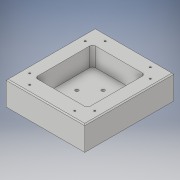
# Autodesk Inventor part: Chuck
Saved by Autodesk Inventor 2019.4 (Build 234330000, 330)
## iProperties
Created: 2020-11-12
Part Number: Chuck
Material: Generic
Document SubType Name: Modeling
Designer: caleb
Density: 1 g/cm^3
Appearance: Default
Author: caleb
Autodesk Inventor part; units mm, degrees
ref_plane "YZ Plane" through (0, 0, 0) normal (1, 0, 0) x (0, 1, 0)
ref_plane "XZ Plane" through (0, 0, 0) normal (0, 1, 0) x (-1, 0, 0)
ref_plane "XY Plane" through (0, 0, 0) normal (0, 0, 1) x (1, 0, 0)
sketch "Sketch1" plane through (0, 0, 0) normal (0, 1, 0) x (-1, 0, 0)
  line L0 (75, 85) -> (-75, 85)
  line L1 (-75, 85) -> (-75, -85)
  line L2 (-75, -85) -> (75, -85)
  line L3 (75, -85) -> (75, 85)
  point P0 (0, 0)
  dimension "d0" = 170
  dimension "d1" = 150
  dimension "d8" = 85
  dimension "d9" = 75
  constraints: 8 end point, 2 parallel, 1 horizontal, 1 perpendicular
  measures "d0" distance of L2.end L0.start
  measures "d1" distance of L0.start L0.end
  measures "d8" distance from line of L0 point (0, 0)
  measures "d9" distance from line of L3 point (0, 0)
extrude "Extrusion1" add sketch "Sketch1" along normal blind 46
sketch "Sketch2" plane through (0, 46, 0) normal (0, 1, 0) x (1, 0, 0)
  line L0 (-50, -55) -> (50, -55)
  line L1 (50, -55) -> (50, 55)
  line L2 (50, 55) -> (-50, 55)
  line L3 (-50, 55) -> (-50, -55)
  point P0 (0, 0)
  dimension "d4" = 100
  dimension "d5" = 110
  dimension "d6" = 55
  dimension "d7" = 50
  constraints: 8 end point, 2 parallel, 1 horizontal, 1 perpendicular
  measures "d4" distance of L0.start L0.end
  measures "d5" distance of L2.end L0.start
  measures "d6" distance from line of L0 point (0, 0)
  measures "d7" distance from line of L3 point (0, 0)
extrude "Extrusion2" cut sketch "Sketch2" against normal blind 36
fillet "Fillet1" radius 5 1 edges at (-50, 28, -55)
fillet "Fillet2" radius 5 1 edges at (-50, 28, 55)
fillet "Fillet3" radius 5 1 edges at (50, 28, 55)
fillet "Fillet4" radius 5 1 edges at (50, 28, -55)
chamfer "Chamfer1" distance 2 angle 45 4 edges at (75, 46, 0) (0, 46, -85) (0, 46, 85) (-75, 46, 0)
sketch "Sketch3" plane through (0, 46, 0) normal (0, 1, 0) x (1, 0, 0)
  circle A0 centre (43, -72) radius 2
  line L0 (73, -83) -> (-73, -83) projected
  line L1 (73, 83) -> (73, -83) projected
  circle A1 centre (62, -53) radius 2
  circle A2 centre (43, 72) radius 2
  circle A3 centre (62, 53) radius 2
  circle A4 centre (-43, -72) radius 2
  circle A5 centre (-62, -53) radius 2
  circle A6 centre (-43, 72) radius 2
  circle A7 centre (-62, 53) radius 2
  point P0 (0, 0)
  point P1 (-73, 83)
  dimension "d19" = 4
  dimension "d20" = 11
  dimension "d21" = 30
  dimension "d22" = 4
  dimension "d23" = 11
  dimension "d24" = 30
  constraints: 8 centre point
  measures "d19" diameter of A0
  measures "d20" distance from line of L0 A0.centre
  measures "d21" distance from line of L1 A0.centre
  measures "d22" diameter of A1
  measures "d23" distance from line of L1 A1.centre
  measures "d24" distance from line of L0 A1.centre
hole "Hole1" at (43, 46, -72) at (62, 46, -53) at (62, 46, 53) at (43, 46, 72) at (-43, 46, 72) at (-62, 46, 53) at (-62, 46, -53) at (-43, 46, -72) direction (0, -1, 0) diameter 3.242 depth 11.8 tip angle 118 thread size "M4x0.7" class "6H" standard "ISO Metric profile"
sketch "Sketch4" plane through (0, 10, 0) normal (0, 1, 0) x (1, 0, 0)
  circle A0 centre (-25, 0) radius 3
  circle A1 centre (0, 25) radius 3
  circle A2 centre (25, 0) radius 3
  circle A3 centre (0, -25) radius 3
  point P0 (0, 0)
  dimension "d32" = 6
  dimension "d34" = 25
  dimension "d35" = 6
  dimension "d36" = 6
  dimension "d37" = 6
  dimension "d39" = 25
  dimension "d40" = 25
  dimension "d42" = 25
  constraints: 4 centre point, 2 horizontal alignment, 2 vertical alignment
  measures "d32" diameter of A0
  measures "d34" distance of point (0, 0) A0.centre
  measures "d35" diameter of A1
  measures "d36" diameter of A2
  measures "d37" diameter of A3
  measures "d39" distance of A3.centre point (0, 0)
  measures "d40" distance of point (0, 0) A1.centre
  measures "d42" distance of point (0, 0) A2.centre
hole "Hole2" at (-25, 10, 0) at (0, 10, -25) at (25, 10, 0) at (0, 10, 25) direction (0, -1, 0) diameter 6 end through all
body "Solid1"
